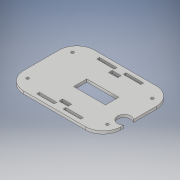
# Autodesk Inventor part: top_plate
Saved by Autodesk Inventor 2017 (Build 210142000, 142)
## iProperties
Created: 2017-06-15
Part Number: top_plate
Material: Generic
Document SubType Name: Modeling
Designer: millerid
Density: 1 g/cm^3
Appearance: Default
Author: millerid
Autodesk Inventor part; units mm, degrees
ref_plane "YZ Plane" through (0, 0, 0) normal (1, 0, 0) x (0, 1, 0)
ref_plane "XZ Plane" through (0, 0, 0) normal (0, 1, 0) x (-1, 0, 0)
ref_plane "XY Plane" through (0, 0, 0) normal (0, 0, 1) x (1, 0, 0)
sketch "Sketch3" plane through (0, 0, 0) normal (0, 1, 0) x (-1, 0, 0)
  line L0 (20, 0) -> (89.97, 0)
  line L1 (109.97, -20) -> (109.97, -60)
  line L2 (89.97, -80) -> (20, -80)
  arc A0 (109.97, -20) -> (89.97, 0) centre (89.97, -20) ccw
  arc A1 (89.97, -80) -> (109.97, -60) centre (89.97, -60) ccw
  arc A2 (0, -60) -> (20, -80) centre (20, -60) ccw
  arc A3 (20, 0) -> (0, -20) centre (20, -20) ccw
  line L3 (79.7968, -4.5) -> (60, -4.5)
  line L4 (60, -4.5) -> (60, -7.4718)
  line L5 (60, -7.4718) -> (79.7968, -7.4718)
  line L6 (79.7968, -7.4718) -> (79.7968, -4.5)
  line L7 (30, -4.5) -> (49.7968, -4.5)
  line L8 (49.7968, -4.5) -> (49.7968, -7.4718)
  line L9 (49.7968, -7.4718) -> (30, -7.4718)
  line L10 (30, -7.4718) -> (30, -4.5)
  line L11 (79.7968, -72.5282) -> (60, -72.5282)
  line L12 (60, -72.5282) -> (60, -75.5)
  line L13 (60, -75.5) -> (79.7968, -75.5)
  line L14 (79.7968, -75.5) -> (79.7968, -72.5282)
  line L15 (49.7968, -72.5282) -> (30, -72.5282)
  line L16 (30, -72.5282) -> (30, -75.5)
  line L17 (30, -75.5) -> (49.7968, -75.5)
  line L18 (49.7968, -75.5) -> (49.7968, -72.5282)
  line L19 (60, -10) -> (49.7968, -10)
  line L20 (49.7968, -10) -> (49.7968, -14)
  line L21 (49.7968, -14) -> (60, -14)
  line L22 (60, -14) -> (60, -10)
  line L23 (49.7968, -70) -> (60, -70)
  line L24 (60, -70) -> (60, -66)
  line L25 (60, -66) -> (49.7968, -66)
  line L26 (49.7968, -66) -> (49.7968, -70)
  circle A4 centre (9.9, -65.4) radius 1.5
  circle A5 centre (100.07, -65.4) radius 1.5
  circle A6 centre (9.9, -14.6) radius 1.5
  circle A7 centre (100.07, -14.6) radius 1.5
  line L27 (65.97, -32.5) -> (29.97, -32.5)
  line L28 (29.97, -32.5) -> (29.97, -47.5)
  line L29 (29.97, -47.5) -> (65.97, -47.5)
  line L30 (65.97, -47.5) -> (65.97, -32.5)
  arc A8 (0, -34.278) -> (0, -22.922) centre (4.9, -28.6) ccw
  line L31 (0, -60) -> (0, -34.278)
  line L32 (0, -22.922) -> (0, -20)
  point P0 (0, 0)
  point P1 (109.97, -80)
  point P2 (109.97, 0)
  point P3 (0, -80)
  dimension "d0" = 109.97
  dimension "d1" = 80
  dimension "d2" = 20
  dimension "d3" = 19.7968
  dimension "d4" = 2.9718
  dimension "d5" = 4.5
  dimension "d7" = 19.7968
  dimension "d9" = 2.9718
  dimension "d10" = 4.5
  dimension "d11" = 4
  dimension "d12" = 10
  dimension "d13" = 4
  dimension "d14" = 10
  dimension "d15" = 3
  dimension "d16" = 3
  dimension "d17" = 3
  dimension "d22" = 9.9
  dimension "d23" = 9.9
  dimension "d26" = 14.6
  dimension "d27" = 14.6
  dimension "d28" = 14.6
  dimension "d29" = 14.6
  dimension "d30" = 36
  dimension "d31" = 15
  dimension "d32" = 44
  dimension "d33" = 32.5
  dimension "d36" = 10.2032
  constraints: 66 end point, 15 parallel, 12 collinear, 11 point on circle, 9 centre point, 8 horizontal, 8 perpendicular, 7 point on line, 6 tangent, 3 equal radius, 1 vertical
  measures "d0" distance of point (109.97, -80) point (0, -80)
  measures "d1" distance of point (109.97, 0) point (109.97, -80)
  measures "d2" radius of A0
  measures "d3" distance of L5.end L4.end
  measures "d4" distance of L4.end L3.end
  measures "d5" distance between parallel lines of L0 L3
  measures "d7" distance of L8.end L9.end
  measures "d9" distance of L12.end L11.end
  measures "d10" distance between parallel lines of L2 L13
  measures "d11" distance of L20.end L19.end
  measures "d12" distance between parallel lines of L0 L19
  measures "d13" distance of L24.end L23.end
  measures "d14" distance between parallel lines of L2 L23
  measures "d15" diameter of A4
  measures "d16" diameter of A5
  measures "d17" diameter of A6
  measures "d22" distance from line of L1 A7.centre
  measures "d23" distance from line of L1 A5.centre
  measures "d26" distance from line of L0 A7.centre
  measures "d27" distance from line of L2 A5.centre
  measures "d28" distance from line of L0 A6.centre
  measures "d29" distance from line of L2 A4.centre
  measures "d30" distance of L29.end L28.end
  measures "d31" distance of L28.end L27.end
  measures "d32" distance between parallel lines of L1 L30
  measures "d33" distance between parallel lines of L0 L27
  measures "d36" distance between parallel lines of L8 L4
extrude "Extrusion1" add sketch "Sketch3" along normal blind 3.175
equation "\"d3\" = d7"
equation "\"d9\" = d4"
equation "\"d10\" = d5"
equation "\"d14\" = d12"
equation "\"d23\" = d22"
equation "\"d27\" = d26"
equation "\"d28\" = d26"
equation "\"d29\" = d26"
equation "\"d33\" = -0.5 * d31 + 0.5 * d1"
body "Solid1"
